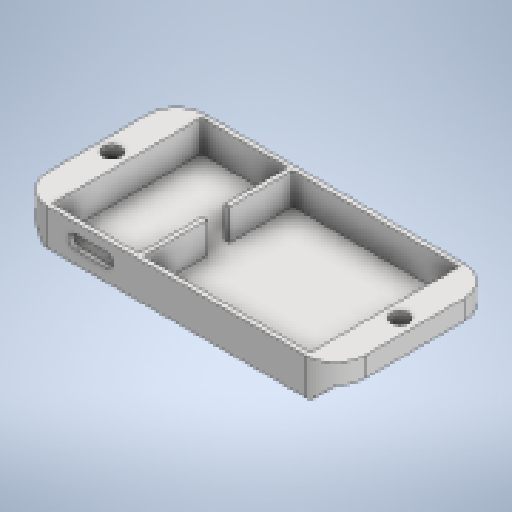
# Autodesk Inventor part: rama
Saved by Autodesk Inventor 2024.3 (Build 283343000, 343)
## iProperties
Created: 2025-07-27
Part Number: rama
Material: Ogólny
Document SubType Name: Modeling
Designer: User
Density: 1 g/cm^3
Appearance: Domyślna
Author: User
Autodesk Inventor part; units mm, degrees
ref_plane "YZ Plane" through (0, 0, 0) normal (1, 0, 0) x (0, 1, 0)
ref_plane "XZ Plane" through (0, 0, 0) normal (0, 1, 0) x (-1, 0, 0)
ref_plane "XY Plane" through (0, 0, 0) normal (0, 0, 1) x (1, 0, 0)
sketch "Szkic1" plane through (0, 0, 0) normal (0, 1, 0) x (-1, 0, 0)
  line L0 (0, 0) -> (52, 0)
  line L1 (52, 0) -> (52, -30)
  line L2 (52, -30) -> (0, -30)
  line L3 (0, -30) -> (0, 0)
  line L4 (-1, 1) -> (53, 1)
  line L5 (53, 1) -> (53, -31)
  line L6 (53, -31) -> (-1, -31)
  line L7 (-1, -31) -> (-1, 1)
  line L8 (-1, 1) -> (53, -31) construction
  line L9 (53, 1) -> (-1, -31) construction
  point P0 (26, -15)
  dimension "d0" = 52
  dimension "d1" = 30
  dimension "d2" = 54
  dimension "d3" = 32
  constraints: 20 end point, 4 parallel, 2 horizontal, 2 midpoint, 2 perpendicular
  measures "d0" distance of L1.end L2.end
  measures "d1" distance of L0.end L1.end
  measures "d2" distance of L5.end L6.end
  measures "d3" distance of L4.end L5.end
extrude "Wyciągnięcie proste1" add sketch "Szkic1" along normal blind 1 contours L0 L1 L2 L3 | L4 L5 L6 L7
extrude "Wyciągnięcie proste2" add sketch "Szkic1" along normal blind 2
sketch "Szkic2" plane through (0, 1, 0) normal (0, 1, 0) x (1, 0, 0)
  line L0 (-52, 30) -> (-52, 0) projected
  line L1 (-52, 15) -> (-34.6, 15)
  line L2 (-43.3, 15) -> (-43.3, 0)
  line L3 (0, 0) -> (-52, 0) projected
  line L4 (-43.3, 0) -> (-40.3, 0)
  line L5 (-40.3, 0) -> (-40.3, -2.2641)
  line L6 (-40.3, -2.2641) -> (-43.3, -2.2641)
  line L7 (-43.3, -2.2641) -> (-43.3, 0)
  line L8 (-43.3, 0) -> (-46.3, 0)
  line L9 (-46.3, 0) -> (-46.3, -2.2641)
  line L10 (-46.3, -2.2641) -> (-43.3, -2.2641)
  line L11 (-43.3, -2.2641) -> (-43.3, 0)
  dimension "d8" = 17.4
  dimension "d9" = 3
  dimension "d10" = 3
  constraints: 20 end point, 4 parallel, 3 point on line, 2 midpoint, 2 perpendicular, 1 horizontal, 1 vertical
  measures "d8" distance of L1.start L1.end
  measures "d9" distance of L2.end L4.end
  measures "d10" distance of L2.end L8.end
extrude "Wyciągnięcie proste3" cut sketch "Szkic2" along normal blind 2 contours L3 L7 L10 L9 | L3 L5 L6 L7
sketch "Szkic3" plane through (0, 1, 0) normal (0, 1, 0) x (1, 0, 0)
  line L0 (-52, 0) -> (-52, 30) projected
  line L1 (-52, 15) -> (-34.5, 15)
  line L2 (0, 30) -> (-52, 30) projected
  line L3 (-34.5, 15) -> (-34.5, 30)
  line L4 (-34.5, 30) -> (-33.6, 30)
  line L5 (-33.6, 30) -> (-33.6, 15)
  line L6 (-33.6, 15) -> (-34.5, 15)
  line L7 (-34.5, 15) -> (-34.5, 30)
  line L8 (-34.5, 30) -> (-34.6, 30)
  line L9 (-34.6, 30) -> (-34.6, 15)
  line L10 (-34.6, 15) -> (-34.5, 15)
  line L11 (0, 0) -> (-40.3, 0) projected
  line L12 (-34.6, 30) -> (-34.6, 0)
  line L13 (-34.6, 0) -> (-33.6, 0)
  line L14 (-33.6, 0) -> (-33.6, 30)
  line L15 (-33.6, 30) -> (-34.6, 30)
  point P0 (-33.6, 0)
  dimension "d13" = 17.5
  dimension "d14" = 0.9
  dimension "d15" = 0.1
  dimension "d16" = 1
  constraints: 26 end point, 7 equal length, 3 perpendicular, 3 point on line, 1 horizontal, 1 midpoint, 1 vertical
  measures "d13" distance of L1.start L1.end
  measures "d14" distance of L3.end L4.end
  measures "d15" distance of L8.end L3.end
  measures "d16" distance of L13.end L12.end
extrude "Wyciągnięcie proste4" add sketch "Szkic3" along normal blind 1 contours L9 L2 L3 L1 | L1 L6 L14 L11 L12 | L3 L2 L5 L6
sketch "Szkic4" plane through (0, 1, 0) normal (0, 1, 0) x (1, 0, 0)
  line L0 (-53, 31) -> (-53, -1) projected
  line L1 (-53, 15) -> (1, 15)
  line L2 (1, -1) -> (1, 31) projected
  line L3 (1, 31) -> (-53, 31) projected
  line L4 (-26, 31) -> (-26, -1)
  line L5 (-53, -1) -> (1, -1) projected
  line L6 (-33.6, 0) -> (0, 0) projected
  line L7 (-33.6, 0) -> (-33.6, 30)
  line L8 (0, 15) -> (-31.4, 15)
  line L9 (0, 15) -> (31.4, 15) construction
  line L10 (-34.6, 0) -> (-34.6, 30) projected
  line L11 (-34.6, 15) -> (-31.4, 15)
  circle A0 centre (-33, 15) radius 1.25
  line L12 (0, 30) -> (0, 0) projected
  line L13 (-34.75, 12.75) -> (-31.25, 12.75)
  line L14 (-31.25, 12.75) -> (-31.25, 17.25)
  line L15 (-31.25, 17.25) -> (-34.75, 17.25)
  line L16 (-34.75, 17.25) -> (-34.75, 12.75)
  line L17 (-34.75, 12.75) -> (-31.25, 17.25) construction
  line L18 (-31.25, 12.75) -> (-34.75, 17.25) construction
  line L19 (-34.75, 12.75) -> (-31.25, 12.75)
  line L20 (-31.25, 12.75) -> (-31.25, 17.25)
  line L21 (-31.25, 17.25) -> (-34.75, 17.25)
  line L22 (-34.75, 17.25) -> (-34.75, 12.75)
  line L23 (-34.75, 12.75) -> (-31.25, 17.25) construction
  line L24 (-31.25, 12.75) -> (-34.75, 17.25) construction
  dimension "d20" = 180
  dimension "d21" = 2.5
  dimension "d29" = 33
  dimension "d42" = 3.5
  dimension "d43" = 4.5
  constraints: 36 end point, 11 midpoint, 4 parallel, 3 collinear, 3 horizontal, 2 perpendicular, 1 centre point, 1 point on line
  measures "d20" angle of L8 L9
  measures "d21" diameter of A0
  measures "d29" distance of point (0, 15) A0.centre
  measures "d42" distance of L15.end L14.end
  measures "d43" distance of L14.end L13.end
extrude "Wyciągnięcie proste5" cut sketch "Szkic4" along normal blind 2.25 contours L16 L15 L10 L1 | L1 L10 L13 L16 | L10 L15 L7 A0 L1 | L1 A0 L7 L13 L10 | L14 L13 L7 A0 L1 | L1 A0 L7 L15 L14 | A0 L7 L1 | L1 L7 A0 | L7 A0 L1 | L1 A0 L7
move faces "Przesuń2" translate (0, 5.3, 0) faces at (-28.8667, 2, -30.6667)
sketch "Szkic5" plane through (0, 1, 0) normal (0, 1, 0) x (1, 0, 0)
  line L0 (-46.3, -1) -> (-46.3, 0) projected
  line L1 (-40.3, -1) -> (-46.3, -1) projected
  line L2 (-46.3, -1) -> (-40.3, -1)
  line L3 (-40.3, -1) -> (-40.3, 0)
  line L4 (-40.3, 0) -> (-46.3, 0)
  line L5 (-46.3, 0) -> (-46.3, -1)
  point P0 (0, 0)
  constraints: 8 end point, 2 parallel, 1 horizontal, 1 perpendicular
extrude "Wyciągnięcie proste6" add sketch "Szkic5" along normal blind 1.8
sketch "Szkic6" plane through (-53, 0, 1) normal (0, 0, 1) x (1, 0, 0)
  line L0 (12.7, 2.8) -> (6.7, 2.8) projected
  line L1 (12.7, 2.8) -> (6.7, 2.8)
  line L2 (6.7, 2.8) -> (6.7, 7.3)
  line L3 (1, 7.3) -> (18.4, 7.3) projected
  line L4 (12.8, 3.9) -> (6.6, 3.9) construction
  line L5 (12.8, 5.3) -> (6.6, 5.3)
  line L6 (6.6, 2.5) -> (12.8, 2.5)
  arc A0 (12.8, 2.5) -> (12.8, 5.3) centre (12.8, 3.9) ccw
  arc A1 (6.6, 5.3) -> (6.6, 2.5) centre (6.6, 3.9) ccw
  line L7 (9.7, 3.9) -> (15.9, 3.9) construction
  point P0 (53, 0)
  point P1 (9.7, 7.3)
  dimension "d32" = 3.1
  dimension "d33" = 180
  dimension "d34" = 2.8
  dimension "d37" = 3.4
  constraints: 14 end point, 4 point on circle, 4 tangent, 2 centre point, 2 equal length, 2 midpoint, 2 perpendicular, 1 collinear, 1 horizontal, 1 point on line
  measures "d32" distance of L7.start L4.end
  measures "d33" angle of L4 L7
  measures "d34" diameter of A1
  measures "d37" distance of point (9.7, 7.3) L7.start
extrude "Wyciągnięcie proste7" cut sketch "Szkic6" against normal blind 1.8
sketch "Szkic8" plane through (-40.3, 7.3, 0) normal (-1, 0, 0) x (0, 0, 1)
  line L0 (0, 0) -> (1, 0) projected
  line L1 (0, 0) -> (1, 0)
  line L2 (1, 0) -> (1, -1)
  line L3 (1, -1) -> (0, -1)
  line L4 (0, -1) -> (0, 0)
  point P0 (0, -7.3)
  dimension "d47" = 1
  dimension "d48" = 1
  constraints: 8 end point, 2 parallel, 1 horizontal, 1 perpendicular
  measures "d47" distance of L2.end L3.end
  measures "d48" distance of L1.end L2.end
extrude "Wyciągnięcie proste9" add sketch "Szkic8" along normal blind 9.5
sketch "Szkic9" plane through (-53, 7.3, 1) normal (0, 1, 0) x (1, 0, 0)
  line L0 (54, 0) -> (54, 32) projected
  line L1 (54, 32) -> (59, 32)
  line L2 (59, 32) -> (59, 0)
  line L3 (59, 0) -> (54, 0)
  line L4 (54, 0) -> (54, 32)
  line L5 (0, 0) -> (54, 0) projected
  line L6 (0, 0) -> (-5, 0)
  line L7 (-5, 0) -> (-5, 32)
  line L8 (-5, 32) -> (0, 32)
  line L9 (0, 32) -> (0, 0)
  circle A0 centre (-2, 16) radius 1.8
  circle A1 centre (56, 16) radius 1.8
  circle A2 centre (56, 16) radius 2.05
  circle A3 centre (-2, 16) radius 2.05
  point P0 (53, 1)
  point P1 (0, 16)
  point P2 (0, 15.55)
  point P3 (0, 16.45)
  point P4 (54, 16.45)
  point P5 (54, 15.55)
  dimension "d51" = 5
  dimension "d52" = 32
  dimension "d53" = 5
  dimension "d54" = 32
  dimension "d55" = 3.6
  dimension "d56" = 3.6
  dimension "d64" = 2
  dimension "d65" = 2
  dimension "d73" = 4.1
  dimension "d74" = 4.1
  constraints: 16 end point, 4 centre point, 4 parallel, 2 coincident, 2 horizontal, 2 perpendicular, 1 midpoint
  measures "d51" distance of L2.end L3.end
  measures "d52" distance of L1.end L2.end
  measures "d53" distance of L7.end L8.end
  measures "d54" distance of L6.end L7.end
  measures "d55" diameter of A0
  measures "d56" diameter of A1
  measures "d64" distance of A0.centre point (0, 16)
  measures "d65" distance from line of A1.centre L0
  measures "d73" diameter of A2
  measures "d74" diameter of A3
extrude "Wyciągnięcie proste10" add sketch "Szkic9" against normal blind 4 contours L0 A2 L1 L2 L3 | L0 A2 | L6 L7 L8 L9 A3 | A3 L9 picked at (54.0667, 16) picked at (-0.0667, 16)
fillet "Zaokrąglenie1" radius 6 4 edges at (-58, 5.3, 1) (-58, 5.3, -31) (6, 5.3, 1) (6, 5.3, -31)
move faces "Przesuń3" translate (0, -1, 0) faces at (-44.3, 6.3, 0.6667)
sketch "Szkic11" plane through (0, 0, 0) normal (0, -1, 0) x (1, 0, 0)
  line L0 (-14.8351, -24.201) -> (-2.0509, -24.201) construction
  line L1 (-2.0509, -24.201) -> (-2.0509, -38.9677) construction
  line L2 (-2.0509, -38.9677) -> (-14.8351, -38.9677) construction
  line L3 (-14.8351, -38.9677) -> (-14.8351, -24.201) construction
  spline S0 degree 2 poles (-10.9372, -27.7545) (-10.9372, -28.1272) (-11.2208, -28.6985) (-11.4558, -28.8849) knots 0 0 0 1 2 2 2
  spline S1 degree 2 poles (-11.4558, -28.8849) (-11.7394, -29.1037) (-12.3837, -29.2901) (-12.8942, -29.2901) knots 0 0 0 1 2 2 2
  line L4 (-12.8942, -29.2901) -> (-14.3286, -29.2901)
  line L5 (-14.3286, -29.2901) -> (-14.3286, -24.2901)
  line L6 (-14.3286, -24.2901) -> (-13.0036, -24.2901)
  spline S2 degree 2 poles (-13.0036, -24.2901) (-12.4688, -24.2901) (-11.9339, -24.359) (-11.6908, -24.4927) knots 0 0 0 1 2 2 2
  spline S3 degree 2 poles (-11.6908, -24.4927) (-11.4193, -24.6345) (-11.1722, -25.1005) (-11.1722, -25.4165) knots 0 0 0 1 2 2 2
  spline S4 degree 2 poles (-11.1722, -25.4165) (-11.1722, -25.769) (-11.5449, -26.3282) (-11.8731, -26.4862) knots 0 0 0 1 2 2 2
  line L7 (-11.8731, -26.4862) -> (-11.8731, -26.5105)
  spline S5 degree 2 poles (-11.8731, -26.5105) (-11.4274, -26.6321) (-10.9372, -27.2763) (-10.9372, -27.7545) knots 0 0 0 1 2 2 2
  spline S6 degree 2 poles (-11.63, -27.7828) (-11.63, -27.4992) (-11.7921, -27.1345) (-12.0352, -27.0049) knots 0 0 0 1 2 2 2
  spline S7 degree 2 poles (-12.0352, -27.0049) (-12.1932, -26.9238) (-12.566, -26.8752) (-12.9104, -26.8752) knots 0 0 0 1 2 2 2
  line L8 (-12.9104, -26.8752) -> (-13.6641, -26.8752)
  line L9 (-13.6641, -26.8752) -> (-13.6641, -28.7228)
  line L10 (-13.6641, -28.7228) -> (-13.1252, -28.7228)
  spline S8 degree 2 poles (-13.1252, -28.7228) (-12.6876, -28.7228) (-12.1851, -28.6418) (-11.9906, -28.5121) knots 0 0 0 1 2 2 2
  spline S9 degree 2 poles (-11.9906, -28.5121) (-11.8043, -28.3784) (-11.63, -28.0462) (-11.63, -27.7828) knots 0 0 0 1 2 2 2
  spline S10 degree 2 poles (-11.865, -25.5097) (-11.865, -25.3314) (-11.9866, -25.064) (-12.1203, -24.987) knots 0 0 0 1 2 2 2
  spline S11 degree 2 poles (-12.1203, -24.987) (-12.2824, -24.8979) (-12.6754, -24.8574) (-13.0279, -24.8574) knots 0 0 0 1 2 2 2
  line L11 (-13.0279, -24.8574) -> (-13.6641, -24.8574)
  line L12 (-13.6641, -24.8574) -> (-13.6641, -26.3201)
  line L13 (-13.6641, -26.3201) -> (-12.9104, -26.3201)
  spline S12 degree 2 poles (-12.9104, -26.3201) (-12.5984, -26.3201) (-12.3026, -26.2553) (-12.1446, -26.154) knots 0 0 0 1 2 2 2
  spline S13 degree 2 poles (-12.1446, -26.154) (-11.9906, -26.0567) (-11.865, -25.7447) (-11.865, -25.5097) knots 0 0 0 1 2 2 2
  line L14 (-9.3448, -29.2901) -> (-10.147, -29.2901)
  line L15 (-10.147, -29.2901) -> (-10.147, -28.3339)
  line L16 (-10.147, -28.3339) -> (-9.3448, -28.3339)
  line L17 (-9.3448, -28.3339) -> (-9.3448, -29.2901)
  spline S14 degree 2 poles (-6.8002, -29.3792) (-7.3432, -29.3792) (-8.1049, -29.1523) (-8.4412, -28.9903) knots 0 0 0 1 2 2 2
  line L18 (-8.4412, -28.9903) -> (-8.4412, -28.1556)
  line L19 (-8.4412, -28.1556) -> (-8.3926, -28.1556)
  spline S15 degree 2 poles (-8.3926, -28.1556) (-8.0644, -28.4635) (-7.2338, -28.8039) (-6.8488, -28.8039) knots 0 0 0 1 2 2 2
  spline S16 degree 2 poles (-6.8488, -28.8039) (-6.2978, -28.8039) (-5.7346, -28.346) (-5.7346, -27.9692) knots 0 0 0 1 2 2 2
  spline S17 degree 2 poles (-5.7346, -27.9692) (-5.7346, -27.6694) (-6.0304, -27.2966) (-6.3505, -27.2034) knots 0 0 0 1 2 2 2
  spline S18 degree 2 poles (-6.3505, -27.2034) (-6.5814, -27.1386) (-6.9663, -27.0494) (-7.254, -26.9765) knots 0 0 0 1 2 2 2
  spline S19 degree 2 poles (-7.254, -26.9765) (-7.5133, -26.9076) (-7.9226, -26.701) (-8.0806, -26.5348) knots 0 0 0 1 2 2 2
  spline S20 degree 2 poles (-8.0806, -26.5348) (-8.2346, -26.3687) (-8.4047, -25.923) (-8.4047, -25.6313) knots 0 0 0 1 2 2 2
  spline S21 degree 2 poles (-8.4047, -25.6313) (-8.4047, -25.0235) (-7.4566, -24.201) (-6.7232, -24.201) knots 0 0 0 1 2 2 2
  spline S22 degree 2 poles (-6.7232, -24.201) (-6.3018, -24.201) (-5.5563, -24.3671) (-5.2362, -24.5251) knots 0 0 0 1 2 2 2
  line L20 (-5.2362, -24.5251) -> (-5.2362, -25.3193)
  line L21 (-5.2362, -25.3193) -> (-5.2848, -25.3193)
  spline S23 degree 2 poles (-5.2848, -25.3193) (-5.5239, -25.1005) (-6.2694, -24.7763) (-6.6787, -24.7763) knots 0 0 0 1 2 2 2
  spline S24 degree 2 poles (-6.6787, -24.7763) (-7.1406, -24.7763) (-7.7119, -25.2099) (-7.7119, -25.5624) knots 0 0 0 1 2 2 2
  spline S25 degree 2 poles (-7.7119, -25.5624) (-7.7119, -25.8784) (-7.3756, -26.2553) (-7.0595, -26.3404) knots 0 0 0 1 2 2 2
  spline S26 degree 2 poles (-7.0595, -26.3404) (-6.8488, -26.3971) (-6.237, -26.5429) (-6.0344, -26.6037) knots 0 0 0 1 2 2 2
  spline S27 degree 2 poles (-6.0344, -26.6037) (-5.5198, -26.7617) (-5.0417, -27.3979) (-5.0417, -27.8639) knots 0 0 0 1 2 2 2
  spline S28 degree 2 poles (-5.0417, -27.8639) (-5.0417, -28.1596) (-5.2808, -28.7269) (-5.4955, -28.9254) knots 0 0 0 1 2 2 2
  spline S29 degree 2 poles (-5.4955, -28.9254) (-5.7346, -29.1442) (-6.3423, -29.3792) (-6.8002, -29.3792) knots 0 0 0 1 2 2 2
  line L22 (-3.4331, -29.2901) -> (-4.2354, -29.2901)
  line L23 (-4.2354, -29.2901) -> (-4.2354, -28.3339)
  line L24 (-4.2354, -28.3339) -> (-3.4331, -28.3339)
  line L25 (-3.4331, -28.3339) -> (-3.4331, -29.2901)
  point P0 (0, 0)
  constraints: 2 other
extrude "Wyciągnięcie proste11" cut sketch "Szkic11" against normal blind 0.4
extrude "Wyciągnięcie proste12" cut sketch "Szkic9" against normal blind 1 contours L0 A2 | A3 L9 picked at (54.0667, 16) picked at (-0.0667, 16)
